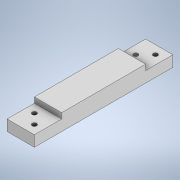
# Autodesk Inventor part: Axel_crossbar_final
Saved by Autodesk Inventor 2020 (Build 240168000, 168)
## iProperties
Created: 2022-06-14
Part Number: Axel_crossbar_final
Material: 일반
Document SubType Name: Modeling
Designer: samsung
Density: 1 g/cm^3
Appearance: 기본값
Author: samsung
Autodesk Inventor part; units mm, degrees
ref_plane "YZ Plane" through (0, 0, 0) normal (1, 0, 0) x (0, 1, 0)
ref_plane "XZ Plane" through (0, 0, 0) normal (0, 1, 0) x (-1, 0, 0)
ref_plane "XY Plane" through (0, 0, 0) normal (0, 0, 1) x (1, 0, 0)
sketch "스케치1" plane through (0, 0, 0) normal (0, 0, 1) x (1, 0, 0)
  line L0 (0, 0) -> (25, 0)
  line L1 (25, 0) -> (25, 15)
  line L2 (25, 15) -> (0, 15)
  line L3 (0, 15) -> (0, 0)
  dimension "d0" = 25
  dimension "d1" = 15
  constraints: 8 end point, 2 parallel, 1 horizontal, 1 perpendicular
  measures "d0" distance of L2.end L1.end
  measures "d1" distance of L1.end L0.end
extrude "돌출1" add sketch "스케치1" against normal blind 127
sketch "스케치2" plane through (25, 0, 0) normal (1, 0, 0) x (0, 0, -1)
  line L0 (0, 0) -> (0, 15) projected
  line L1 (0, 0) -> (127, 0) projected
  line L2 (127, 15) -> (127, 0) projected
  line L3 (0, 15) -> (127, 15) projected
  line L4 (0, 15) -> (25, 15)
  line L5 (25, 15) -> (25, 10)
  line L6 (25, 10) -> (0, 10)
  line L7 (0, 10) -> (0, 15)
  line L8 (127, 15) -> (102, 15)
  line L9 (102, 15) -> (102, 10)
  line L10 (102, 10) -> (127, 10)
  line L11 (127, 10) -> (127, 15)
  dimension "d4" = 25
  dimension "d5" = 5
  dimension "d6" = 25
  dimension "d7" = 5
  constraints: 16 end point, 4 parallel, 2 horizontal, 2 perpendicular
  measures "d4" distance of L5.end L6.end
  measures "d5" distance of L4.end L5.end
  measures "d6" distance of L10.end L9.end
  measures "d7" distance of L9.end L8.end
extrude "돌출2" cut sketch "스케치2" against normal blind 127 contours L0 L3 L5 L6 | L10 L9 L3 L2
sketch "스케치3" plane through (25, 10, 0) normal (0, 1, 0) x (1, 0, 0)
  line L0 (-25, 0) -> (-25, 25) projected
  line L1 (0, 0) -> (-25, 0) projected
  line L2 (0, 25) -> (0, 0) projected
  line L3 (0, 25) -> (-25, 25) projected
  line L4 (-25, 102) -> (-25, 127) projected
  line L5 (0, 102) -> (-25, 102) projected
  line L6 (0, 127) -> (0, 102) projected
  line L7 (-25, 127) -> (0, 127) projected
  point P0 (-8, 8)
  point P1 (-17, 17)
  point P2 (-17, 110)
  point P3 (-8, 119)
  dimension "d10" = 8
  dimension "d11" = 8
  dimension "d12" = 8
  dimension "d13" = 8
  dimension "d14" = 8
  dimension "d15" = 8
  dimension "d16" = 8
  dimension "d17" = 8
  measures "d10" distance from line of L1 point (-8, 8)
  measures "d11" distance from line of L2 point (-8, 8)
  measures "d12" distance from line of L3 point (-17, 17)
  measures "d13" distance from line of L0 point (-17, 17)
  measures "d14" distance from line of L4 point (-17, 110)
  measures "d15" distance from line of L5 point (-17, 110)
  measures "d16" distance from line of L6 point (-8, 119)
  measures "d17" distance from line of L7 point (-8, 119)
hole "구멍1" at (17, 10, -8) at (8, 10, -17) at (8, 10, -110) at (17, 10, -119) direction (0, -1, 0) diameter 4.134 end through all thread size "M5x0.8" class "6H" standard "ISO Metric profile"
